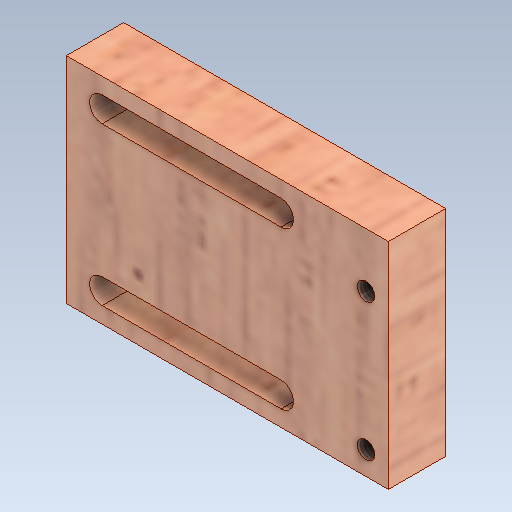
# Autodesk Inventor part: 0005-10-021 suport senzor z
Saved by Autodesk Inventor 2020 (Build 240168000, 168)
## iProperties
Created: 2020-12-18
Part Number: 0005-10-021 suport senzor z
Material: Generic
Document SubType Name: Modeling
Designer: Iulian Bors
Density: 1 g/cm^3
Appearance: White Oak - Natural Medium Gloss
Mass: 9.17008 g
Surface Area: 45.9205 cm^2
Volume: 9.17008 cm^3
Author: Iulian Bors
Subject: 021
Autodesk Inventor part; units mm, degrees
ref_plane "YZ Plane" through (0, 0, 0) normal (1, 0, 0) x (0, 1, 0)
ref_plane "XZ Plane" through (0, 0, 0) normal (0, 1, 0) x (-1, 0, 0)
ref_plane "XY Plane" through (0, 0, 0) normal (0, 0, 1) x (1, 0, 0)
sketch "Sketch1" plane through (0, 0, 0) normal (0, 0, 1) x (1, 0, 0)
  line L0 (-22.5, 15) -> (22.5, 15)
  line L1 (22.5, 15) -> (22.5, -15)
  line L2 (22.5, -15) -> (-22.5, -15)
  line L3 (-22.5, -15) -> (-22.5, 15)
  point P0 (0, 0)
  point P1 (0, 15)
  point P2 (-22.5, 0)
  dimension "d0" = 45
  dimension "d1" = 30
  constraints: 8 end point, 2 midpoint, 2 parallel, 1 horizontal, 1 horizontal alignment, 1 perpendicular, 1 vertical alignment
  measures "d0" distance of L0.start L0.end
  measures "d1" distance of L2.end L0.start
extrude "Extrusion1" add sketch "Sketch1" along normal blind 8
sketch "Sketch5" plane through (0, 0, 8) normal (0, 0, 1) x (1, 0, 0)
  line L0 (7.5, 11) -> (-17.5, 11) construction
  line L1 (7.5, 12.75) -> (-17.5, 12.75)
  line L2 (-17.5, 9.25) -> (7.5, 9.25)
  arc A0 (7.5, 9.25) -> (7.5, 12.75) centre (7.5, 11) ccw
  arc A1 (-17.5, 12.75) -> (-17.5, 9.25) centre (-17.5, 11) ccw
  line L3 (7.5, -11) -> (-17.5, -11) construction
  line L4 (7.5, -9.25) -> (-17.5, -9.25)
  line L5 (-17.5, -12.75) -> (7.5, -12.75)
  arc A2 (7.5, -12.75) -> (7.5, -9.25) centre (7.5, -11) ccw
  arc A3 (-17.5, -9.25) -> (-17.5, -12.75) centre (-17.5, -11) ccw
  line L6 (22.5, 15) -> (-22.5, 15) projected
  line L7 (-22.5, -15) -> (22.5, -15) projected
  line L8 (-22.5, 15) -> (-22.5, -15) projected
  point P0 (0, 0)
  point P1 (-5, 11)
  point P2 (-5, -11)
  dimension "d29" = 3.5
  dimension "d30" = 4
  dimension "d31" = 4
  dimension "d33" = 25
  dimension "d36" = 5
  constraints: 16 end point, 8 point on circle, 8 tangent, 5 parallel, 4 centre point, 2 midpoint, 1 equal radius, 1 horizontal, 1 vertical alignment
  measures "d29" distance between parallel lines of L2 L1
  measures "d30" distance between parallel lines of L0 L6
  measures "d31" distance between parallel lines of L7 L3
  measures "d33" distance of L0.start L0.end
  measures "d36" distance from line of L8 L0.end
extrude "Extrusion5" cut sketch "Sketch5" against normal blind 10
sketch "Sketch6" plane through (0, 0, 8) normal (0, 0, 1) x (1, 0, 0)
  circle A0 centre (19.3725, -11.7625) radius 1.7875 projected
  circle A1 centre (19.3725, 7.4125) radius 1.7875 projected
  point P0 (0, 0)
hole "Hole1" at (19.3725, 7.4125, 8) at (19.3725, -11.7625, 8) direction (0, 0, -1) diameter 2.459 end through all thread size "M3x0.5" class "6H" standard "ISO Metric profile"
body "Solid1"
